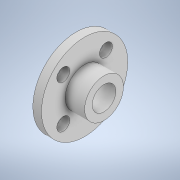
# Autodesk Inventor part: ServoHornRound
Saved by Autodesk Inventor 2020 (Build 240168000, 168)
## iProperties
Created: 2023-12-31
Part Number: ServoHornRound
Material: Generic
Document SubType Name: Modeling
Designer: smz3rm
Density: 1 g/cm^3
Appearance: Default
Author: smz3rm
Autodesk Inventor part; units mm, degrees
ref_plane "YZ Plane" through (0, 0, 0) normal (1, 0, 0) x (0, 1, 0)
ref_plane "XZ Plane" through (0, 0, 0) normal (0, 1, 0) x (-1, 0, 0)
ref_plane "XY Plane" through (0, 0, 0) normal (0, 0, 1) x (1, 0, 0)
sketch "Sketch1" plane through (0, 0, 0) normal (1, 0, 0) x (0, 1, 0)
  circle A0 centre (0, 0) radius 10
  circle A1 centre (4.9497, 4.9497) radius 1.5
  circle A2 centre (4.9497, -4.9497) radius 1.5
  circle A3 centre (-4.9497, 4.9497) radius 1.5
  circle A4 centre (-4.9497, -4.9497) radius 1.5
  line L0 (4.9497, 4.9497) -> (4.9497, -4.9497)
  line L1 (4.9497, -4.9497) -> (-4.9497, -4.9497)
  line L2 (-4.9497, -4.9497) -> (-4.9497, 4.9497)
  line L3 (-4.9497, 4.9497) -> (4.9497, 4.9497)
  line L4 (4.9497, 0) -> (0, 0)
  line L5 (4.9497, 4.9497) -> (-4.9497, -4.9497)
  circle A5 centre (0, 0) radius 1.5
  dimension "d0" = 20
  dimension "d1" = 3
  dimension "d2" = 3
  dimension "d3" = 3
  dimension "d4" = 3
  dimension "d7" = 14
  dimension "d10" = 3
  constraints: 12 end point, 6 centre point, 3 coincident, 2 horizontal, 2 midpoint, 2 parallel, 1 perpendicular, 1 vertical
  measures "d0" diameter of A0
  measures "d1" diameter of A1
  measures "d2" diameter of A2
  measures "d3" diameter of A3
  measures "d4" diameter of A4
  measures "d7" distance of L0.start L1.end
  measures "d10" diameter of A5
extrude "Extrusion1" add sketch "Sketch1" along normal blind 2 contours A0 | A1 L5 A5 A4 L2 A3 L3 | L0 L4 A5 L5 A1 | L0 A2 L1 A4 L5 A5 L4
sketch "Sketch2" plane through (2, 0, 0) normal (1, 0, 0) x (0, 0, -1)
  circle A0 centre (0, 0) radius 2.75
  circle A1 centre (0, 0) radius 4.5
  dimension "d11" = 5.5
  dimension "d12" = 9
  constraints: 2 centre point, 2 coincident
  measures "d11" diameter of A0
  measures "d12" diameter of A1
extrude "Extrusion2" add sketch "Sketch2" along normal blind 4.5
body "Solid1"
